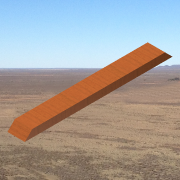
# Autodesk Inventor part: 2p2ps45
Saved by Autodesk Inventor 2013 SP2 (Build 170200200, 200)
## iProperties
Company: HERA Project
Created: 2013-09-03
Part Number: 2p2ps45
Material: Wood (Cherry)
Document SubType Name: Modeling
Designer: David DeBoer
Mass: 1214.71 g
Surface Area: 1927.86 cm^2
Volume: 2429.41 cm^3
Density: 0.5 g/cm^3
Description: pole stand support 45 degree
Author: David DeBoer
Autodesk Inventor part; units mm, degrees
ref_plane "YZ Plane" through (0, 0, 0) normal (1, 0, 0) x (0, 1, 0)
ref_plane "XZ Plane" through (0, 0, 0) normal (0, 1, 0) x (-1, 0, 0)
ref_plane "XY Plane" through (0, 0, 0) normal (0, 0, 1) x (1, 0, 0)
sketch "Sketch1" plane through (0, 0, 0) normal (1, 0, 0) x (0, 1, 0)
  line L0 (38.1, -38.1) -> (38.1, -717.55)
  line L1 (0, -755.65) -> (0, 0)
  line L2 (0, 0) -> (38.1, -38.1)
  line L3 (0, 0) -> (78.5772, 0) construction
  line L4 (0, -755.65) -> (38.1, -717.55)
  dimension "d2" = 45
  dimension "d20" = 755.65
  constraints: 10 end point, 1 horizontal, 1 parallel, 1 perpendicular
  measures "d2" angle of L2 L3
  measures "d20" distance of L1.start L1.end
extrude "Extrusion1" add sketch "Sketch1" along normal blind 88.9
sketch "Sketch2" plane through (88.9, 38.1, -717.55) normal (0, 0.7071, -0.7071) x (-1, 0, 0)
  line L0 (0, -53.8815) -> (0, 0) projected
  line L1 (88.9, -53.8815) -> (0, -53.8815) projected
  circle A0 centre (25.4, -26.9408) radius 4.5233
  circle A1 centre (63.5, -26.9408) radius 4.5233
  point P0 (88.9, 480.4437)
  dimension "d5" = 25.4
  dimension "d8" = 38.1
  constraints: 2 centre point, 1 horizontal, 2 other
  measures "d5" distance from line of L0 A0.centre
  measures "d8" distance of A0.centre A1.centre
hole "Hole1" at (63.5, 19.05, -736.6) at (25.4, 19.05, -736.6) direction (0, -0.7071, 0.7071) diameter 6.35 depth 25.4 tip angle 118
body "Solid1"
